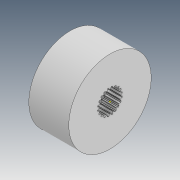
# Autodesk Inventor part: roda certa 2.0
Saved by Autodesk Inventor 2021 (Build 250183000, 183)
## iProperties
Created: 2020-10-21
Part Number: roda certa 2.0
Material: Genérico
Document SubType Name: Modeling
Designer: evert
Density: 1 g/cm^3
Appearance: Padrão
Author: evert
Autodesk Inventor part; units mm, degrees
ref_plane "YZ Plane" through (0, 0, 0) normal (1, 0, 0) x (0, 1, 0)
ref_plane "XZ Plane" through (0, 0, 0) normal (0, 1, 0) x (-1, 0, 0)
ref_plane "XY Plane" through (0, 0, 0) normal (0, 0, 1) x (1, 0, 0)
sketch "Esboço2" plane through (0, 0, 0) normal (0, 0, 1) x (1, 0, 0)
  line L0 (0, 0) -> (9.5, 0)
  line L1 (9.5, 0) -> (9.5, 9.8)
  line L2 (9.5, 9.8) -> (0, 9.8)
  line L3 (0, 9.8) -> (0, 0)
  dimension "d0" = 9.5
  dimension "d1" = 9.8
  constraints: 8 end point, 2 parallel, 1 horizontal, 1 perpendicular
  measures "d0" distance of L1.end L2.end
  measures "d1" distance of L0.end L1.end
revolve "Revolução1" add sketch "Esboço2" angle 360 about axis through (0, 0, 0) along (1, 0, 0)
sketch "Esboço3" plane through (0, 0, 0) normal (-1, 0, 0) x (0, 0, 1)
  circle A0 centre (0, 0) radius 1.75
  dimension "d3" = 3.5
  constraints: 1 centre point, 1 coincident
  measures "d3" diameter of A0
extrude "Extrusão1" cut sketch "Esboço3" against normal blind 4.85
sketch "Esboço4" plane through (0, 0, 0) normal (-1, 0, 0) x (0, 0, 1)
  circle A0 centre (0, 0) radius 4.5
  dimension "d6" = 9
  constraints: 1 centre point, 1 coincident
  measures "d6" diameter of A0
extrude "Extrusão2" cut sketch "Esboço4" against normal blind 2
sketch "Esboço11" plane through (9.5, 0, 0) normal (1, 0, 0) x (0, 0, -1)
  circle A0 centre (0, 0) radius 2.55
  circle A1 centre (0, 0) radius 2.95
  line L0 (0, 0) -> (2.95, 0)
  line L1 (2.55, 0) -> (2.5493, 0.06)
  line L2 (2.5493, 0.06) -> (2.55, 0)
  line L3 (2.55, 0) -> (2.5493, -0.06)
  line L4 (2.5493, 0.06) -> (2.9315, 0.3295)
  line L5 (2.5493, -0.06) -> (2.9315, -0.3295)
  line L6 (2.9315, 0.3295) -> (2.9255, 0.3791)
  line L7 (2.9315, -0.3295) -> (2.9255, -0.3791)
  line L8 (2.406, 0.8448) -> (2.6862, 1.2193)
  line L9 (2.4252, 0.788) -> (2.406, 0.8448)
  line L10 (2.4252, 0.788) -> (2.4431, 0.7307)
  line L11 (2.4431, 0.7307) -> (2.8899, 0.5925)
  circle A2 centre (0, 0) radius 2.95
  line L12 (2.6862, 1.2193) -> (2.6652, 1.2646)
  line L13 (2.8899, 0.5925) -> (2.8995, 0.5435)
  line L14 (2.0272, 1.547) -> (2.178, 1.9897)
  line L15 (2.063, 1.4989) -> (2.0272, 1.547)
  line L16 (2.063, 1.4989) -> (2.0977, 1.4499)
  line L17 (2.0977, 1.4499) -> (2.5653, 1.4566)
  circle A3 centre (0, 0) radius 2.95
  line L18 (2.178, 1.9897) -> (2.144, 2.0263)
  line L19 (2.5653, 1.4566) -> (2.5897, 1.4129)
  line L20 (1.4499, 2.0977) -> (1.4566, 2.5653)
  line L21 (1.4989, 2.063) -> (1.4499, 2.0977)
  line L22 (1.4989, 2.063) -> (1.547, 2.0272)
  line L23 (1.547, 2.0272) -> (1.9897, 2.178)
  circle A4 centre (0, 0) radius 2.95
  line L24 (1.4566, 2.5653) -> (1.4129, 2.5897)
  line L25 (1.9897, 2.178) -> (2.0263, 2.144)
  line L26 (0.7307, 2.4431) -> (0.5925, 2.8899)
  line L27 (0.788, 2.4252) -> (0.7307, 2.4431)
  line L28 (0.788, 2.4252) -> (0.8448, 2.406)
  line L29 (0.8448, 2.406) -> (1.2193, 2.6862)
  circle A5 centre (0, 0) radius 2.95
  line L30 (0.5925, 2.8899) -> (0.5435, 2.8995)
  line L31 (1.2193, 2.6862) -> (1.2646, 2.6652)
  line L32 (-0.06, 2.5493) -> (-0.3295, 2.9315)
  line L33 (0, 2.55) -> (-0.06, 2.5493)
  line L34 (0, 2.55) -> (0.06, 2.5493)
  line L35 (0.06, 2.5493) -> (0.3295, 2.9315)
  circle A6 centre (0, 0) radius 2.95
  line L36 (-0.3295, 2.9315) -> (-0.3791, 2.9255)
  line L37 (0.3295, 2.9315) -> (0.3791, 2.9255)
  line L38 (-0.8448, 2.406) -> (-1.2193, 2.6862)
  line L39 (-0.788, 2.4252) -> (-0.8448, 2.406)
  line L40 (-0.788, 2.4252) -> (-0.7307, 2.4431)
  line L41 (-0.7307, 2.4431) -> (-0.5925, 2.8899)
  circle A7 centre (0, 0) radius 2.95
  line L42 (-1.2193, 2.6862) -> (-1.2646, 2.6652)
  line L43 (-0.5925, 2.8899) -> (-0.5435, 2.8995)
  line L44 (-1.547, 2.0272) -> (-1.9897, 2.178)
  line L45 (-1.4989, 2.063) -> (-1.547, 2.0272)
  line L46 (-1.4989, 2.063) -> (-1.4499, 2.0977)
  line L47 (-1.4499, 2.0977) -> (-1.4566, 2.5653)
  circle A8 centre (0, 0) radius 2.95
  line L48 (-1.9897, 2.178) -> (-2.0263, 2.144)
  line L49 (-1.4566, 2.5653) -> (-1.4129, 2.5897)
  line L50 (-2.0977, 1.4499) -> (-2.5653, 1.4566)
  line L51 (-2.063, 1.4989) -> (-2.0977, 1.4499)
  line L52 (-2.063, 1.4989) -> (-2.0272, 1.547)
  line L53 (-2.0272, 1.547) -> (-2.178, 1.9897)
  circle A9 centre (0, 0) radius 2.95
  line L54 (-2.5653, 1.4566) -> (-2.5897, 1.4129)
  line L55 (-2.178, 1.9897) -> (-2.144, 2.0263)
  line L56 (-2.4431, 0.7307) -> (-2.8899, 0.5925)
  line L57 (-2.4252, 0.788) -> (-2.4431, 0.7307)
  line L58 (-2.4252, 0.788) -> (-2.406, 0.8448)
  line L59 (-2.406, 0.8448) -> (-2.6862, 1.2193)
  circle A10 centre (0, 0) radius 2.95
  line L60 (-2.8899, 0.5925) -> (-2.8995, 0.5435)
  line L61 (-2.6862, 1.2193) -> (-2.6652, 1.2646)
  line L62 (-2.5493, -0.06) -> (-2.9315, -0.3295)
  line L63 (-2.55, 0) -> (-2.5493, -0.06)
  line L64 (-2.55, 0) -> (-2.5493, 0.06)
  line L65 (-2.5493, 0.06) -> (-2.9315, 0.3295)
  circle A11 centre (0, 0) radius 2.95
  line L66 (-2.9315, -0.3295) -> (-2.9255, -0.3791)
  line L67 (-2.9315, 0.3295) -> (-2.9255, 0.3791)
  line L68 (-2.406, -0.8448) -> (-2.6862, -1.2193)
  line L69 (-2.4252, -0.788) -> (-2.406, -0.8448)
  line L70 (-2.4252, -0.788) -> (-2.4431, -0.7307)
  line L71 (-2.4431, -0.7307) -> (-2.8899, -0.5925)
  circle A12 centre (0, 0) radius 2.95
  line L72 (-2.6862, -1.2193) -> (-2.6652, -1.2646)
  line L73 (-2.8899, -0.5925) -> (-2.8995, -0.5435)
  line L74 (-2.0272, -1.547) -> (-2.178, -1.9897)
  line L75 (-2.063, -1.4989) -> (-2.0272, -1.547)
  line L76 (-2.063, -1.4989) -> (-2.0977, -1.4499)
  line L77 (-2.0977, -1.4499) -> (-2.5653, -1.4566)
  circle A13 centre (0, 0) radius 2.95
  line L78 (-2.178, -1.9897) -> (-2.144, -2.0263)
  line L79 (-2.5653, -1.4566) -> (-2.5897, -1.4129)
  line L80 (-1.4499, -2.0977) -> (-1.4566, -2.5653)
  line L81 (-1.4989, -2.063) -> (-1.4499, -2.0977)
  line L82 (-1.4989, -2.063) -> (-1.547, -2.0272)
  line L83 (-1.547, -2.0272) -> (-1.9897, -2.178)
  circle A14 centre (0, 0) radius 2.95
  line L84 (-1.4566, -2.5653) -> (-1.4129, -2.5897)
  line L85 (-1.9897, -2.178) -> (-2.0263, -2.144)
  line L86 (-0.7307, -2.4431) -> (-0.5925, -2.8899)
  line L87 (-0.788, -2.4252) -> (-0.7307, -2.4431)
  line L88 (-0.788, -2.4252) -> (-0.8448, -2.406)
  line L89 (-0.8448, -2.406) -> (-1.2193, -2.6862)
  circle A15 centre (0, 0) radius 2.95
  line L90 (-0.5925, -2.8899) -> (-0.5435, -2.8995)
  line L91 (-1.2193, -2.6862) -> (-1.2646, -2.6652)
  line L92 (0.06, -2.5493) -> (0.3295, -2.9315)
  line L93 (0, -2.55) -> (0.06, -2.5493)
  line L94 (0, -2.55) -> (-0.06, -2.5493)
  line L95 (-0.06, -2.5493) -> (-0.3295, -2.9315)
  circle A16 centre (0, 0) radius 2.95
  line L96 (0.3295, -2.9315) -> (0.3791, -2.9255)
  line L97 (-0.3295, -2.9315) -> (-0.3791, -2.9255)
  line L98 (0.8448, -2.406) -> (1.2193, -2.6862)
  line L99 (0.788, -2.4252) -> (0.8448, -2.406)
  line L100 (0.788, -2.4252) -> (0.7307, -2.4431)
  line L101 (0.7307, -2.4431) -> (0.5925, -2.8899)
  circle A17 centre (0, 0) radius 2.95
  line L102 (1.2193, -2.6862) -> (1.2646, -2.6652)
  line L103 (0.5925, -2.8899) -> (0.5435, -2.8995)
  line L104 (1.547, -2.0272) -> (1.9897, -2.178)
  line L105 (1.4989, -2.063) -> (1.547, -2.0272)
  line L106 (1.4989, -2.063) -> (1.4499, -2.0977)
  line L107 (1.4499, -2.0977) -> (1.4566, -2.5653)
  circle A18 centre (0, 0) radius 2.95
  line L108 (1.9897, -2.178) -> (2.0263, -2.144)
  line L109 (1.4566, -2.5653) -> (1.4129, -2.5897)
  line L110 (2.0977, -1.4499) -> (2.5653, -1.4566)
  line L111 (2.063, -1.4989) -> (2.0977, -1.4499)
  line L112 (2.063, -1.4989) -> (2.0272, -1.547)
  line L113 (2.0272, -1.547) -> (2.178, -1.9897)
  circle A19 centre (0, 0) radius 2.95
  line L114 (2.5653, -1.4566) -> (2.5897, -1.4129)
  line L115 (2.178, -1.9897) -> (2.144, -2.0263)
  line L116 (2.4431, -0.7307) -> (2.8899, -0.5925)
  line L117 (2.4252, -0.788) -> (2.4431, -0.7307)
  line L118 (2.4252, -0.788) -> (2.406, -0.8448)
  line L119 (2.406, -0.8448) -> (2.6862, -1.2193)
  circle A20 centre (0, 0) radius 2.95
  line L120 (2.8899, -0.5925) -> (2.8995, -0.5435)
  line L121 (2.6862, -1.2193) -> (2.6652, -1.2646)
  point P0 (2.8056, 0.9116)
  point P1 (2.3866, 1.734)
  point P2 (1.734, 2.3866)
  point P3 (0.9116, 2.8056)
  point P4 (0, 2.95)
  point P5 (-0.9116, 2.8056)
  point P6 (-1.734, 2.3866)
  point P7 (-2.3866, 1.734)
  point P8 (-2.8056, 0.9116)
  point P9 (-2.95, 0)
  point P10 (-2.8056, -0.9116)
  point P11 (-2.3866, -1.734)
  point P12 (-1.734, -2.3866)
  point P13 (-0.9116, -2.8056)
  point P14 (0, -2.95)
  point P15 (0.9116, -2.8056)
  point P16 (1.734, -2.3866)
  point P17 (2.3866, -1.734)
  point P18 (2.8056, -0.9116)
  dimension "d59" = 5.9
  dimension "d58" = 5.1
  dimension "d60" = 0.06
  dimension "d61" = 0.06
  dimension "d62" = 0.05
  dimension "d63" = 0.05
  dimension "d66" = 360
  constraints: 244 end point, 98 point on circle, 20 centre point, 4 coincident, 2 coincident with centre, 1 collinear, 1 horizontal, 1 point on line, 324 other
  measures "d58" diameter of A0
  measures "d60" distance of L1.start L1.end
  measures "d61" distance of L1.start L3.end
  measures "d62" distance of L4.end L6.end
  measures "d63" distance of L5.end L7.end
extrude "Extrusão5" cut sketch "Esboço11" against normal blind 3.5 contours A0 | A0 L11 A1 L4 | L5 A1 L116 A0 | A0 L17 A1 L8 | L119 A1 L110 A0 | A0 L23 A1 L14 | L113 A1 L104 A0 | A0 L29 A1 L20 | L107 A1 L98 A0 | A0 L35 A1 L26 | L101 A1 L92 A0 | A0 L41 A1 L32 | L95 A1 L86 A0 | A0 L47 A1 L38 | L89 A1 L80 A0 | A0 L53 A1 L44 | L83 A1 L74 A0 | A0 L59 A1 L50 | L77 A1 L68 A0 | A0 L65 A1 L56 | L71 A1 L62 A0
sketch "Esboço12" plane through (9.5, 0, 0) normal (1, 0, 0) x (0, 0, -1)
  point P0 (0, 0)
